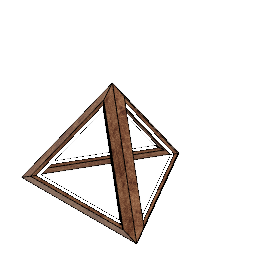
TetraHedral tale Lamp v2 (Autodesk Fusion 360 design; units mm, degrees)
Autodesk Fusion 360 part; units mm, degrees
sketch "Sketch1" plane through (0, 0, 0) normal (0, 0, 1) x (1, 0, 0)
  line L0 (0, 0) -> (10, 0)
  line L1 (10, 0) -> (0, 17.3205)
  line L2 (0, 17.3205) -> (-10, 0)
  line L3 (-10, 0) -> (0, 0)
  dimension "d1" = 60
  dimension "d2" = 20
  constraint coincident L0.start L3.end
  constraint horizontal L0
  constraint parallel L0 L3
  measures "d1" angle of L0 L1
  measures "d2" distance of L0.end L1.end
sketch "Sketch2" plane through (0, 0, 0) normal (1, 0, 0) x (0, 1, 0)
  line L0 (0, 0) -> (0, 0.5)
  line L1 (0, 0.5) -> (0.866, 0)
  line L2 (0, 0.5) -> (1, 0.5) construction
  line L3 (0.866, 0) -> (0, -0.5)
  line L4 (0, -0.5) -> (0, 0)
  line L5 (0, 0.5) -> (-3.7, 0.5)
  line L6 (0, -0.5) -> (-1.4134, 0.5)
  line L7 (0.45, 0.2402) -> (0.45, -0.2402)
  dimension "d3" = 30
  dimension "d4" = 1
  dimension "d5" = 54.72
  dimension "d6" = 0.45
  constraint coincident L0.start L4.end
  constraint vertical L0
  constraint horizontal L2
  constraint parallel L0 L4
  constraint perpendicular L0 L5
  constraint coincident L5 L6.end
  constraint coincident L1 L7.start
  constraint coincident L3 L7.end
  constraint perpendicular L2 L7
  measures "d3" angle of L1 L2
  measures "d4" distance of L0.end L1.end
  measures "d5" angle of L4 L6
  measures "d6" distance of L0 L7
sweep "Sweep1" add profiles "Sketch2" path "Sketch1" along L0 L1 L2 L3 section 1 contours L0 L4 L5 L6 | L0 L1 L3 L4 L7 makes body 1
sweep "Sweep2" add profiles "Sketch2" path "Sketch1" along L2 L3 L0 L1 section 1 contours L1 L3 L7 separate body makes body 2
copy_body "CopyPasteBodies1" bodies 1 2 makes body 3 makes body 4
move_body "Move1" bodies 3 4 to x (1, 0, 0) y (0, 0.333807, -0.942641) z (0, 0.942641, 0.333807) at (0, -1.4129, -0.9992)
copy_body "CopyPasteBodies2" bodies 1 2 makes body 5 makes body 6
move_body "Move2" bodies 5 6 to x (0.500355, 0.28847, -0.816351) y (0.28847, 0.833452, 0.471321) z (0.816351, -0.471321, 0.333807) at (-6.2201, 3.5912, -9.1627)
move_body "Move4" bodies 2 1 to x (0.500355, -0.28847, 0.816351) y (-0.28847, 0.833452, 0.471321) z (-0.816351, -0.471321, 0.333807) at (6.2201, 3.5912, -9.1627)
move_body "Move5" bodies 1 2 3 4 5 6 to x (-1, 0, 0) y (0, 1, 0) z (0, 0, -1) at (-0.0177, 0, -39.648)
move_body "Move6" bodies 1 2 3 4 5 6 to x (1, 0, 0) y (0, 1, 0) z (0, 0, 1) at (0, 0, 40)
